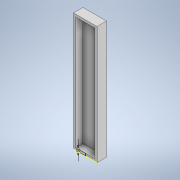
# Autodesk Inventor part: S.hollow box
Saved by Autodesk Inventor 2020 (Build 240168000, 168)
## iProperties
Created: 2020-04-13
Part Number: S.hollow box
Material: Generic
Document SubType Name: Modeling
Designer: Darugar
Density: 1 g/cm^3
Appearance: Default
Author: Darugar
Autodesk Inventor part; units mm, degrees
ref_plane "YZ Plane" through (0, 0, 0) normal (1, 0, 0) x (0, 1, 0)
ref_plane "XZ Plane" through (0, 0, 0) normal (0, 1, 0) x (-1, 0, 0)
ref_plane "XY Plane" through (0, 0, 0) normal (0, 0, 1) x (1, 0, 0)
sketch "Sketch1" plane through (0, 0, 0) normal (0, 0, 1) x (1, 0, 0)
  line L0 (0, 0) -> (100, 0)
  line L1 (100, 0) -> (100, 500)
  line L2 (100, 500) -> (0, 500)
  line L3 (0, 500) -> (0, 0)
  dimension "d0" = 100
  dimension "d1" = 500
  constraints: 8 end point, 2 parallel, 1 horizontal, 1 perpendicular
  measures "d0" distance of L2.end L1.end
  measures "d1" distance of L1.end L0.end
extrude "Extrusion1" add sketch "Sketch1" along normal blind 40
sketch "Sketch2" plane through (0, 0, 40) normal (0, 0, 1) x (1, 0, 0)
  line L0 (0, 0) -> (100, 0) projected
  line L1 (50, 0) -> (50, 10)
  dimension "d4" = 10
  constraints: 2 end point, 1 midpoint, 1 vertical
  measures "d4" distance of L1.start L1.end
sketch "Sketch3" plane through (0, 0, 40) normal (0, 0, 1) x (1, 0, 0)
  line L0 (100, 500) -> (0, 500) projected
  line L1 (50, 500) -> (50, 490)
  line L2 (100, 0) -> (100, 500) projected
  line L3 (100, 250) -> (90, 250)
  line L4 (0, 500) -> (0, 0) projected
  line L5 (0, 250) -> (10, 250)
  line L6 (90, 490) -> (10, 490)
  line L7 (10, 490) -> (10, 9.7366)
  line L8 (10, 9.7366) -> (90, 9.7366)
  line L9 (90, 9.7366) -> (90, 490)
  dimension "d5" = 10
  dimension "d7" = 10
  constraints: 14 end point, 3 horizontal, 3 midpoint, 2 parallel, 1 perpendicular, 1 vertical
  measures "d5" distance of L1.start L1.end
  measures "d7" distance of L5.start L5.end
extrude "Extrusion2" cut sketch "Sketch3" against normal blind 30 contours L6 L9 L8 L7
body "Solid1"
